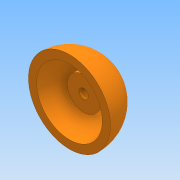
# Autodesk Inventor part: Ball_Upper Half
Saved by Autodesk Inventor 2018.1 (Build 221171000, 171)
## iProperties
Created: 2019-02-18
Part Number: Ball_Upper Half
Material: Nylon 6/6
Document SubType Name: Modeling
Designer: James
Density: 1.13 g/cm^3
Appearance: Orange
Author: James
Autodesk Inventor part; units mm, degrees
ref_plane "YZ Plane" through (0, 0, 0) normal (1, 0, 0) x (0, 1, 0)
ref_plane "XY Plane" through (0, 0, 0) normal (0, 0, 1) x (1, 0, 0)
sketch "Sketch1" plane through (0, 0, 0) normal (0, 0, 1) x (1, 0, 0)
  line L0 (0, 0) -> (0, 20)
  line L1 (0, 0) -> (20, 0)
  arc A0 (20, 0) -> (0, 20) centre (0, 0) ccw
  line L2 (0, -4.8284) -> (0, 28.9706) projected
  dimension "d2" = 20
  constraints: 4 end point, 2 coincident, 2 point on circle, 1 centre point, 1 horizontal, 1 vertical
  measures "d2" distance of L0.start L0.end
revolve "Revolution1" add sketch "Sketch1" angle 360 about axis through (0, -10, 0) along (0, 1, 0)
ref_plane "Work Plane1" through (0, 15, 0) normal (0, 1, 0) x (-1, 0, 0)
sketch "Sketch2" plane through (0, 15, 0) normal (0, 1, 0) x (-1, 0, 0)
  point P0 (0, 0)
  point P1 (0, 0)
  constraints: 1 coincident
hole "Hole1" at (0, 15, 0) direction (0, -1, 0) diameter 4.5 end through all counterbore diameter 8 counterbore depth 4 clearance for "Socket Head Cap Screw" size "M4" standard "Ansi Metric M Profile"
shell "Shell1" thickness 4 removed faces 1 at (13.8841, 0, 1.6858)
sketch "Sketch3" plane through (0, 0, 0) normal (0, -1, 0) x (1, 0, 0)
  circle A0 centre (0, 0) radius 6.25 projected
  circle A1 centre (0, 0) radius 2.25 projected
extrude "Extrusion1" cut sketch "Sketch3" against normal blind 7
body "Solid1"
